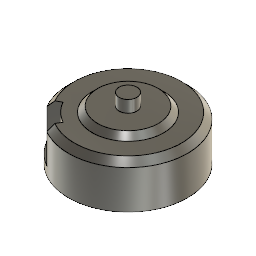
Base prototype (Autodesk Fusion 360 design; units mm, degrees)
Autodesk Fusion 360 part; units mm, degrees
sketch "Sketch1" plane through (0, 0, 0) normal (0, 0, 1) x (1, 0, 0)
  circle A0 centre (0, 0) radius 100
  dimension "d1" = 200
  measures "d1" diameter of A0
extrude "Extrude1" add sketch "Sketch1" along normal blind 75
chamfer "Chamfer1" distance 10 angle 45 1 edges at (-93.2327, -36.1615, 75)
sketch "Sketch2" plane through (0, 0, 75) normal (0, 0, 1) x (-1, 0, 0)
  circle A0 centre (0, 0) radius 90
  circle A1 centre (0, 0) radius 100
  line L0 (0, 0) -> (0, 100)
  line L1 (0, 0) -> (100, 0)
  circle A2 centre (0, 0) radius 80
  line L2 (0, 0) -> (100, 0)
  line L3 (0, 0) -> (139.8681, 80.7529)
  line L4 (0, 0) -> (161.5058, 0) construction
  line L5 (0, 0) -> (61.5265, 106.567)
  dimension "d5" = 160
  dimension "d6" = 30
  dimension "d7" = 60
  measures "d5" diameter of A2
  measures "d6" angle of L3 L4
  measures "d7" angle of L4 L5
extrude "Extrude2" cut sketch "Sketch2" against normal blind 60 contours A0 A2 L3 L5 | A0 A1 L3 L5
sketch "Sketch3" plane through (0, 0, 75) normal (0, 0, 1) x (-1, 0, 0)
  line L0 (40, 69.282) -> (45, 77.9423)
  arc A0 (45, 77.9423) -> (77.9423, 45) centre (0, 0) ccw
  line L1 (77.9423, 45) -> (69.282, 40)
  arc A1 (69.282, 40) -> (40, 69.282) centre (0, 0) ccw
  circle A2 centre (0, 0) radius 60
  dimension "d11" = 120
  measures "d11" diameter of A2
extrude "Extrude3" add sketch "Sketch3" along normal blind 9 draft -45 contours A2
sketch "Sketch4" plane through (0, 0, 84) normal (0, 0, 1) x (-1, 0, 0)
  circle A0 centre (0, 0) radius 51
  circle A1 centre (0, 0) radius 15
  dimension "d14" = 30
  measures "d14" diameter of A1
extrude "Extrude4" add sketch "Sketch4" along normal blind 20 contours A1
